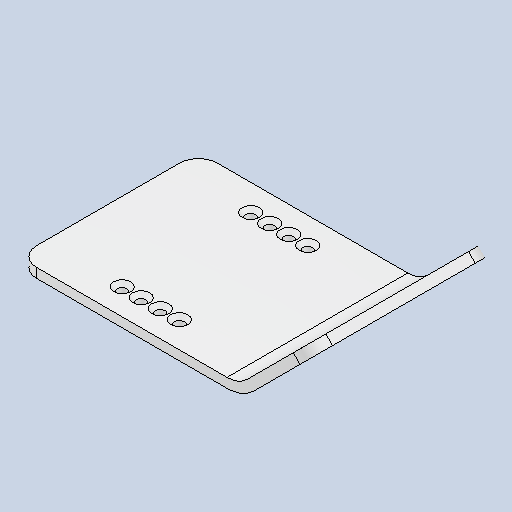
# Autodesk Inventor part: Ramp
Saved by Autodesk Inventor 2023.2 (Build 272271000, 271)
## iProperties
Created: 2024-01-21
Part Number: Ramp
Material: Aluminum 6061
Document SubType Name: Modeling
Designer: Nathan Cai
Mass: 57.3541 g
Surface Area: 147.204 cm^2
Volume: 21.2423 cm^3
Density: 2.7 g/cm^3
Appearance: Aluminum - Flat
Author: Nathan Cai
Autodesk Inventor part; units mm, degrees
ref_plane "YZ Plane" through (0, 0, 0) normal (1, 0, 0) x (0, 1, 0)
ref_plane "XZ Plane" through (0, 0, 0) normal (0, 1, 0) x (-1, 0, 0)
ref_plane "XY Plane" through (0, 0, 0) normal (0, 0, 1) x (1, 0, 0)
sketch "Sketch1" plane through (0, 0, 0) normal (0, 1, 0) x (-1, 0, 0)
  line L0 (-53.975, 30.1625) -> (53.975, 30.1625)
  line L1 (53.975, 30.1625) -> (53.975, -30.1625)
  line L2 (53.975, -30.1625) -> (-53.975, -30.1625)
  line L3 (-53.975, -30.1625) -> (-53.975, 30.1625)
  line L4 (-53.975, 30.1625) -> (53.975, -30.1625) construction
  line L5 (53.975, 30.1625) -> (-53.975, -30.1625) construction
  line L6 (-15.875, -30.1625) -> (-15.875, 30.1625)
  line L7 (-28.575, -12.7) -> (-79.375, -12.7) construction
  line L8 (-79.375, -12.7) -> (-79.375, 12.7)
  line L9 (-79.375, 12.7) -> (-28.575, 12.7) construction
  line L10 (-28.575, 12.7) -> (-28.575, -12.7)
  line L11 (-28.575, -12.7) -> (-79.375, 12.7) construction
  line L12 (-79.375, -12.7) -> (-28.575, 12.7) construction
  line L13 (-28.575, -12.7) -> (-53.975, -19.5059)
  line L14 (-79.375, 0) -> (-28.575, 0) construction
  line L15 (-28.575, 12.7) -> (-53.975, 19.5059)
  point P0 (0, 0)
  point P1 (-53.975, 0)
  point P2 (-53.975, 19.5059)
  dimension "d0" = 107.95
  dimension "d1" = 60.325
  dimension "d11" = 69.85
  dimension "d18" = 50.8
  dimension "d19" = 25.4
  dimension "d20" = 15
  constraints: 32 end point, 7 midpoint, 4 parallel, 3 point on line, 2 horizontal, 2 perpendicular, 1 symmetric about line, 1 vertical
  measures "d0" distance of L1.end L2.end
  measures "d1" distance of L0.end L1.end
  measures "d11" distance between parallel lines of L1 L6
  measures "d18" distance of L8.end L9.end
  measures "d19" distance of L7.end L8.end
  measures "d20" angle of L7 L13
extrude "Extrusion1" add sketch "Sketch1" along normal blind 3.175
bend part "Bend Part1" radius 12.7 angle 45 line through (15.875, 0, -30.1625) along (0, 0, 1) centre toward (0, 1, 0) moving side (1, 0, 0) both sides no
fillet "Fillet1" radius 6.35 4 edges at (43.6204, 24.73, 30.1625) (43.6204, 24.73, -30.1625) (-53.975, 1.5875, -30.1625) (-53.975, 1.5875, 30.1625)
sketch "Sketch3" plane through (0, 3.175, 0) normal (0, 1, 0) x (1, 0, 0)
  point P0 (-8.778, 21.4313)
  point P1 (-15.128, 21.4313)
  point P2 (-21.478, 21.4313)
  point P3 (-27.828, 21.4313)
  point P4 (-8.778, -21.4312)
  point P5 (-15.128, -21.4312)
  point P6 (-21.478, -21.4312)
  point P7 (-27.828, -21.4312)
hole "Hole2" at (-8.778, 3.175, -21.4313) at (-15.128, 3.175, -21.4313) at (-21.478, 3.175, -21.4313) at (-27.828, 3.175, -21.4313) at (-8.778, 3.175, 21.4312) at (-15.128, 3.175, 21.4312) at (-21.478, 3.175, 21.4312) at (-27.828, 3.175, 21.4312) direction (0, -1, 0) diameter 3.2639 end through all countersink diameter 5.715 countersink angle 82
body "Solid1"
